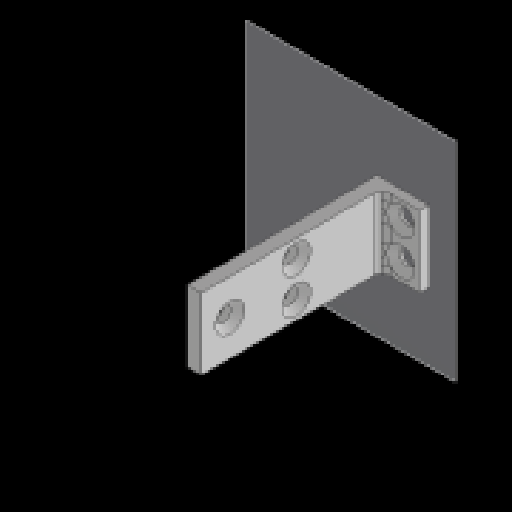
# Autodesk Inventor part: colorSensorHolder2
Saved by Autodesk Inventor 2024.3 (Build 283343010, 343A)
## iProperties
Created: 2025-05-28
Part Number: colorSensorHolder2
Material: Generic
Document SubType Name: Modeling
Designer: Oleg Kelner
Density: 1 g/cm^3
Appearance: Default
Author: Oleg Kelner
Autodesk Inventor part; units mm, degrees
ref_plane "YZ Plane" through (0, 0, 0) normal (1, 0, 0) x (0, 1, 0)
ref_plane "XZ Plane" through (0, 0, 0) normal (0, 1, 0) x (-1, 0, 0)
ref_plane "XY Plane" through (0, 0, 0) normal (0, 0, 1) x (1, 0, 0)
ref_plane "Work Plane1" through (0, 0, 0) normal (0, 0, 1) x (1, 0, 0)
sketch "Sketch1" plane through (0, 0, 0) normal (0, 0, 1) x (1, 0, 0)
  circle A0 centre (0, 0) radius 20 construction
  circle A1 centre (10.45, 12.5) radius 1.75 construction
  circle A2 centre (10.45, -12.5) radius 1.75 construction
  circle A3 centre (-10.45, 12.5) radius 1.75 construction
  circle A4 centre (-10.45, -12.5) radius 1.75 construction
  line L0 (-6.5984, 12.21) -> (-6.5984, 15.25) construction
  line L1 (-6.5984, 15.25) -> (6.6016, 15.25) construction
  line L2 (6.6016, 15.25) -> (6.6016, 12.21) construction
  line L3 (6.6016, 12.21) -> (-6.5984, 12.21) construction
  line L4 (6.6016, -12.21) -> (6.6016, -15.25) construction
  line L5 (6.6016, -15.25) -> (-6.5984, -15.25) construction
  line L6 (-6.5984, -15.25) -> (-6.5984, -12.21) construction
  line L7 (-6.5984, -12.21) -> (6.6016, -12.21) construction
  line L8 (5.5, 7.5) -> (5.5, -7.5)
  line L9 (5.5, -7.5) -> (8.5, -7.5)
  line L10 (8.5, -7.5) -> (8.5, 7.5)
  line L11 (8.5, 7.5) -> (5.5, 7.5)
  line L12 (5.5, 7.5) -> (8.5, -7.5) construction
  line L13 (5.5, -7.5) -> (8.5, 7.5) construction
  line L14 (0, 0) -> (7, 0) construction
  point P0 (0, 0)
  dimension "d0" = 7
  dimension "d1" = 3
  dimension "d2" = 15
  constraints: 14 end point, 2 midpoint, 2 parallel, 1 horizontal, 1 perpendicular, 1 vertical
  measures "d0" distance of L14.start L14.end
  measures "d1" distance between parallel lines of L10 L8
  measures "d2" distance between parallel lines of L9 L11
extrude "Extrusion1" add sketch "Sketch1" along normal blind 40
sketch "Sketch2" plane through (0, 0, 0) normal (0, 0, -1) x (-1, 0, 0)
  line L0 (-5.5, -7.5) -> (-8.5, -7.5) projected
  line L1 (-8.5, 7.5) -> (-5.5, 7.5) projected
  line L2 (-8.5, -7.5) -> (-8.5, 7.5)
  line L3 (-8.5, 7.5) -> (-16.5, 7.5)
  line L4 (-16.5, 7.5) -> (-16.5, -7.5)
  line L5 (-16.5, -7.5) -> (-8.5, -7.5)
  point P0 (0, 0)
  dimension "d5" = 8
  constraints: 8 end point, 2 parallel, 1 perpendicular, 1 vertical
  measures "d5" distance of L3.end L1.start
extrude "Extrusion2" add sketch "Sketch2" against normal blind 2
sketch "Sketch3" plane through (0, 0, 2) normal (0, 0, 1) x (1, 0, 0)
  line L0 (16.5, -7.5) -> (16.5, 7.5) construction
  line L1 (16.5, 7.5) -> (8.5, 7.5) construction
  line L2 (8.5, -7.5) -> (8.5, 7.5) construction
  line L3 (8.5, -7.5) -> (16.5, -7.5) construction
  point P0 (0, 0)
  point P1 (12.5, 3.75)
  point P2 (12.5, -3.75)
  dimension "d9" = 3.75
  dimension "d10" = 4
  dimension "d11" = 3.75
  dimension "d12" = 4
  measures "d9" distance from line of point (12.5, 3.75) L1
  measures "d10" distance from line of L0 point (12.5, 3.75)
  measures "d11" distance from line of L3 point (12.5, -3.75)
  measures "d12" distance from line of L0 point (12.5, -3.75)
hole "Hole1" at (12.5, 3.75, 2) at (12.5, -3.75, 2) direction (0, 0, -1) diameter 3.2 end through all
sketch "Sketch4" plane through (8.5, -7.5, 40) normal (1, 0, 0) x (0, 0, -1)
  line L0 (0, 0) -> (0, 15) projected
  line L1 (38, 0) -> (0, 0) projected
  line L2 (38, 15) -> (0, 15) projected
  point P0 (40, 7.5)
  point P1 (6, 7.5)
  point P2 (20, 3.75)
  point P3 (20, 11.25)
  dimension "d20" = 20
  dimension "d21" = 20
  dimension "d22" = 3.75
  dimension "d23" = 3.75
  dimension "d24" = 7.5
  dimension "d25" = 6
  measures "d20" distance from line of L0 point (20, 11.25)
  measures "d21" distance from line of L0 point (20, 3.75)
  measures "d22" distance from line of L1 point (20, 3.75)
  measures "d23" distance from line of L2 point (20, 11.25)
  measures "d24" distance from line of L2 point (6, 7.5)
  measures "d25" distance from line of L0 point (6, 7.5)
hole "Hole2" at (8.5, 0, 34) at (8.5, -3.75, 20) at (8.5, 3.75, 20) direction (-1, 0, 0) diameter 3.2 end through all countersink diameter 6 countersink angle 90
sketch "Sketch5" plane through (0, 0, 2) normal (0, 0, 1) x (1, 0, 0)
  circle A0 centre (12.5, 3.75) radius 1.6 projected
  circle A1 centre (12.5, -3.75) radius 1.6 projected
  circle A2 centre (12.5, 3.75) radius 3.5
  circle A3 centre (12.5, -3.75) radius 3.5
  point P0 (0, 0)
  dimension "d37" = 7
  dimension "d38" = 7
  constraints: 2 centre point, 2 coincident
  measures "d37" diameter of A2
  measures "d38" diameter of A3
extrude "Extrusion3" cut sketch "Sketch5" against normal blind 0.1
fillet "Fillet2" radius 5 1 edges at (8.5, 0, 2)
body "Solid1"
